Autodesk Fusion 360 part; units mm, degrees
(part 2 of 5)
  spline S372 degree 3 poles (4.7111, -23.5702) (4.7722, -23.6439) (4.9893, -23.6685) (5.5782, -23.6685) knots 0 0 0 0 1 1 1 1
  spline S373 degree 3 poles (5.5782, -23.6685) (6.2377, -23.6685) (6.3816, -23.6488) (6.4743, -23.546) knots 0 0 0 0 1 1 1 1
  spline S374 degree 3 poles (-7.1959, -23.494) (-7.0891, -23.3973) (-7.0889, -23.3561) (-7.1932, -22.9412) knots 0 0 0 0 1 1 1 1
  spline S375 degree 3 poles (-7.1932, -22.9412) (-7.3658, -22.2555) (-7.3564, -22.261) (-8.3356, -22.2838) knots 0 0 0 0 1 1 1 1
  spline S376 degree 3 poles (-8.3356, -22.2838) (-9.3649, -22.3078) (-9.3935, -22.3315) (-9.1564, -22.9655) knots 0 0 0 0 1 1 1 1
  spline S377 degree 3 poles (-9.1564, -22.9655) (-9.0671, -23.2043) (-8.9493, -23.4445) (-8.8946, -23.4991) knots 0 0 0 0 1 1 1 1
  spline S378 degree 3 poles (-8.8946, -23.4991) (-8.7496, -23.6442) (-7.3571, -23.64) (-7.1958, -23.494) knots 0 0 0 0 1 1 1 1
  line L37 (-7.1958, -23.494) -> (-7.1959, -23.494)
  spline S379 degree 3 poles (-9.9736, -23.403) (-9.8682, -23.2865) (-9.8793, -23.2228) (-10.1295, -22.5104) knots 0 0 0 0 1 1 1 1
  spline S380 degree 3 poles (-10.1295, -22.5104) (-10.2776, -22.0885) (-10.4869, -21.4283) (-10.5946, -21.0433) knots 0 0 0 0 1 1 1 1
  spline S381 degree 3 poles (-10.5946, -21.0433) (-10.7023, -20.6583) (-10.8399, -20.2914) (-10.9004, -20.2281) knots 0 0 0 0 1 1 1 1
  spline S382 degree 3 poles (-10.9004, -20.2281) (-10.994, -20.1302) (-11.2635, -20.1058) (-12.6957, -20.0659) knots 0 0 0 0 1 1 1 1
  spline S383 degree 3 poles (-12.6957, -20.0659) (-14.1773, -20.0246) (-14.3919, -20.0322) (-14.4718, -20.1285) knots 0 0 0 0 1 1 1 1
  spline S384 degree 3 poles (-14.4718, -20.1285) (-14.5866, -20.2669) (-14.5722, -20.3045) (-13.7547, -22.0046) knots 0 0 0 0 1 1 1 1
  spline S385 degree 3 poles (-13.7547, -22.0046) (-13.3004, -22.9493) (-13.0832, -23.3288) (-12.9778, -23.3623) knots 0 0 0 0 1 1 1 1
  spline S386 degree 3 poles (-12.9778, -23.3623) (-12.8973, -23.3878) (-12.3588, -23.4307) (-11.781, -23.4576) knots 0 0 0 0 1 1 1 1
  spline S387 degree 3 poles (-11.781, -23.4576) (-10.0405, -23.5385) (-10.0978, -23.5402) (-9.9736, -23.403) knots 0 0 0 0 1 1 1 1
  spline S388 degree 3 poles (-14.1996, -23.1857) (-14.143, -23.08) (-14.2184, -22.8627) (-14.5697, -22.1181) knots 0 0 0 0 1 1 1 1
  spline S389 degree 3 poles (-14.5697, -22.1181) (-14.8124, -21.604) (-15.101, -20.9628) (-15.2112, -20.6933) knots 0 0 0 0 1 1 1 1
  spline S390 degree 3 poles (-15.2112, -20.6933) (-15.4743, -20.0495) (-15.5372, -19.9847) (-15.9461, -19.9363) knots 0 0 0 0 1 1 1 1
  spline S391 degree 3 poles (-15.9461, -19.9363) (-16.4654, -19.8747) (-16.6, -19.7815) (-16.5476, -19.5194) knots 0 0 0 0 1 1 1 1
  spline S392 degree 3 poles (-16.5476, -19.5194) (-16.5238, -19.4006) (-16.4863, -19.2854) (-16.4641, -19.2633) knots 0 0 0 0 1 1 1 1
  spline S393 degree 3 poles (-16.4641, -19.2633) (-16.4419, -19.2412) (-16.0001, -19.221) (-15.4823, -19.2183) knots 0 0 0 0 1 1 1 1
  spline S394 degree 3 poles (-15.4823, -19.2183) (-14.2548, -19.2118) (-14.2482, -19.2065) (-14.5082, -18.4258) knots 0 0 0 0 1 1 1 1
  spline S395 degree 3 poles (-14.5082, -18.4258) (-14.6119, -18.1144) (-14.7295, -17.8393) (-14.7696, -17.8145) knots 0 0 0 0 1 1 1 1
  spline S396 degree 3 poles (-14.7696, -17.8145) (-14.8097, -17.7898) (-15.6499, -17.7301) (-16.6367, -17.6821) knots 0 0 0 0 1 1 1 1
  spline S397 degree 3 poles (-16.6367, -17.6821) (-18.9056, -17.5715) (-18.8123, -17.5261) (-18.3746, -18.5267) knots 0 0 0 0 1 1 1 1
  spline S398 degree 3 poles (-18.3746, -18.5267) (-17.8444, -19.7387) (-17.26, -20.864) (-17.1434, -20.8975) knots 0 0 0 0 1 1 1 1
  spline S399 degree 3 poles (-17.1434, -20.8975) (-17.0815, -20.9152) (-16.8104, -20.9496) (-16.5409, -20.9738) knots 0 0 0 0 1 1 1 1
  spline S400 degree 3 poles (-16.5409, -20.9738) (-15.8303, -21.0378) (-15.6634, -21.1154) (-15.6911, -21.3691) knots 0 0 0 0 1 1 1 1
  spline S401 degree 3 poles (-15.6911, -21.3691) (-15.7208, -21.6402) (-15.7927, -21.7015) (-16.1537, -21.7631) knots 0 0 0 0 1 1 1 1
  spline S402 degree 3 poles (-16.1537, -21.7631) (-16.6452, -21.847) (-16.6576, -21.9608) (-16.2479, -22.631) knots 0 0 0 0 1 1 1 1
  line L38 (-16.2479, -22.631) -> (-15.8919, -23.2134)
  line L39 (-15.8919, -23.2134) -> (-15.5163, -23.2545)
  spline S403 degree 3 poles (-15.5163, -23.2545) (-15.3098, -23.2771) (-14.945, -23.3008) (-14.7057, -23.307) knots 0 0 0 0 1 1 1 1
  spline S404 degree 3 poles (-14.7057, -23.307) (-14.3431, -23.3165) (-14.2588, -23.2963) (-14.1996, -23.1857) knots 0 0 0 0 1 1 1 1
  spline S405 degree 3 poles (-17.102, -22.9718) (-17.059, -22.8365) (-17.5324, -21.8727) (-17.7164, -21.7208) knots 0 0 0 0 1 1 1 1
  spline S406 degree 3 poles (-17.7164, -21.7208) (-17.7629, -21.6824) (-18.1599, -21.6235) (-18.5986, -21.5898) knots 0 0 0 0 1 1 1 1
  spline S407 degree 3 poles (-18.5986, -21.5898) (-19.239, -21.5407) (-19.415, -21.5473) (-19.4912, -21.6235) knots 0 0 0 0 1 1 1 1
  spline S408 degree 3 poles (-19.4912, -21.6235) (-19.6306, -21.7629) (-19.6169, -21.8042) (-19.2605, -22.3212) knots 0 0 0 0 1 1 1 1
  spline S409 degree 3 poles (-19.2605, -22.3212) (-18.7699, -23.0329) (-18.7746, -23.0291) (-18.3356, -23.0569) knots 0 0 0 0 1 1 1 1
  spline S410 degree 3 poles (-18.3356, -23.0569) (-17.272, -23.1244) (-17.1477, -23.1158) (-17.102, -22.9718) knots 0 0 0 0 1 1 1 1
  spline S411 degree 3 poles (-20.085, -22.7052) (-20.0339, -22.6096) (-20.1018, -22.4584) (-20.3884, -22.0305) knots 0 0 0 0 1 1 1 1
  spline S412 degree 3 poles (-20.3884, -22.0305) (-20.5916, -21.7273) (-20.8035, -21.4536) (-20.8592, -21.4224) knots 0 0 0 0 1 1 1 1
  spline S413 degree 3 poles (-20.8592, -21.4224) (-20.915, -21.3912) (-21.3167, -21.3561) (-21.7518, -21.3445) knots 0 0 0 0 1 1 1 1
  spline S414 degree 3 poles (-21.7518, -21.3445) (-22.7883, -21.3168) (-22.836, -21.3702) (-22.3361, -21.9981) knots 0 0 0 0 1 1 1 1
  spline S415 degree 3 poles (-22.3361, -21.9981) (-21.8149, -22.6526) (-21.7425, -22.7033) (-21.2489, -22.7595) knots 0 0 0 0 1 1 1 1
  spline S416 degree 3 poles (-21.2489, -22.7595) (-20.431, -22.8525) (-20.1571, -22.8397) (-20.085, -22.7052) knots 0 0 0 0 1 1 1 1
  spline S417 degree 3 poles (-23.2586, -22.26) (-23.2271, -22.1608) (-23.2597, -22.0505) (-23.3567, -21.9275) knots 0 0 0 0 1 1 1 1
  spline S418 degree 3 poles (-23.3567, -21.9275) (-23.4366, -21.8262) (-23.8688, -21.1996) (-24.3173, -20.5351) knots 0 0 0 0 1 1 1 1
  spline S419 degree 3 poles (-24.3173, -20.5351) (-24.8725, -19.7122) (-25.1802, -19.3178) (-25.282, -19.2986) knots 0 0 0 0 1 1 1 1
  spline S420 degree 3 poles (-25.282, -19.2986) (-25.3642, -19.283) (-25.8252, -19.2171) (-26.3065, -19.152) knots 0 0 0 0 1 1 1 1
  spline S421 degree 3 poles (-26.3065, -19.152) (-26.7877, -19.0869) (-27.2603, -19.0193) (-27.3565, -19.0016) knots 0 0 0 0 1 1 1 1
  spline S422 degree 3 poles (-27.3565, -19.0016) (-27.4814, -18.9787) (-27.5572, -19.0116) (-27.6213, -19.1165) knots 0 0 0 0 1 1 1 1
  spline S423 degree 3 poles (-27.6213, -19.1165) (-27.7025, -19.2494) (-27.6628, -19.3282) (-27.2043, -19.9434) knots 0 0 0 0 1 1 1 1
  spline S424 degree 3 poles (-27.2043, -19.9434) (-26.2552, -21.2168) (-25.7357, -21.7909) (-25.3964, -21.9414) knots 0 0 0 0 1 1 1 1
  spline S425 degree 3 poles (-25.3964, -21.9414) (-25.0384, -22.1001) (-23.8634, -22.389) (-23.5285, -22.4007) knots 0 0 0 0 1 1 1 1
  spline S426 degree 3 poles (-23.5285, -22.4007) (-23.3591, -22.4065) (-23.2944, -22.3728) (-23.2586, -22.26) knots 0 0 0 0 1 1 1 1
  spline S427 degree 3 poles (-18.3724, -20.6471) (-18.3163, -20.5575) (-18.3683, -20.3894) (-18.5996, -19.9121) knots 0 0 0 0 1 1 1 1
  spline S428 degree 3 poles (-18.5996, -19.9121) (-18.7646, -19.5717) (-19.0595, -18.9199) (-19.2549, -18.4637) knots 0 0 0 0 1 1 1 1
  spline S429 degree 3 poles (-19.2549, -18.4637) (-19.499, -17.8936) (-19.6556, -17.6161) (-19.7556, -17.5766) knots 0 0 0 0 1 1 1 1
  spline S430 degree 3 poles (-19.7556, -17.5766) (-19.8356, -17.545) (-20.6729, -17.4756) (-21.6162, -17.4225) knots 0 0 0 0 1 1 1 1
  spline S431 degree 3 poles (-21.6162, -17.4225) (-23.2619, -17.3298) (-23.3369, -17.3312) (-23.4713, -17.4555) knots 0 0 0 0 1 1 1 1
  spline S432 degree 3 poles (-23.4713, -17.4555) (-23.6106, -17.5844) (-23.6096, -17.5883) (-23.2756, -18.2138) knots 0 0 0 0 1 1 1 1
  line L40 (-23.2756, -18.2138) -> (-22.9399, -18.8425)
  line L41 (-22.9399, -18.8425) -> (-23.138, -19.1378)
  spline S433 degree 3 poles (-23.138, -19.1378) (-23.2893, -19.3634) (-23.3917, -19.4415) (-23.5714, -19.4682) knots 0 0 0 0 1 1 1 1
  spline S434 degree 3 poles (-23.5714, -19.4682) (-23.9431, -19.5235) (-23.9843, -19.6738) (-23.7292, -20.0445) knots 0 0 0 0 1 1 1 1
  spline S435 degree 3 poles (-23.7292, -20.0445) (-23.4858, -20.3982) (-23.4696, -20.4032) (-22.2788, -20.4886) knots 0 0 0 0 1 1 1 1
  spline S436 degree 3 poles (-22.2788, -20.4886) (-21.7451, -20.5269) (-21.6317, -20.5163) (-21.5526, -20.421) knots 0 0 0 0 1 1 1 1
  spline S437 degree 3 poles (-21.5526, -20.421) (-21.4724, -20.3244) (-21.4954, -20.2386) (-21.7125, -19.8254) knots 0 0 0 0 1 1 1 1
  spline S438 degree 3 poles (-21.7125, -19.8254) (-22.0273, -19.2265) (-22.0381, -19.019) (-21.7622, -18.8763) knots 0 0 0 0 1 1 1 1
  spline S439 degree 3 poles (-21.7622, -18.8763) (-21.5644, -18.774) (-21.5523, -18.7777) (-21.3568, -19.0003) knots 0 0 0 0 1 1 1 1
  spline S440 degree 3 poles (-21.3568, -19.0003) (-21.246, -19.1265) (-20.9836, -19.535) (-20.7737, -19.9081) knots 0 0 0 0 1 1 1 1
  spline S441 degree 3 poles (-20.7737, -19.9081) (-20.5638, -20.2811) (-20.3446, -20.6075) (-20.2866, -20.6333) knots 0 0 0 0 1 1 1 1
  spline S442 degree 3 poles (-20.2866, -20.6333) (-20.1603, -20.6895) (-19.1029, -20.7825) (-18.7181, -20.7713) knots 0 0 0 0 1 1 1 1
  spline S443 degree 3 poles (-18.7181, -20.7713) (-18.5465, -20.7662) (-18.4182, -20.7202) (-18.3724, -20.6471) knots 0 0 0 0 1 1 1 1
  spline S444 degree 3 poles (-11.2586, -19.227) (-11.1806, -19.1329) (-11.2075, -18.9413) (-11.4286, -18.0142) knots 0 0 0 0 1 1 1 1
  spline S445 degree 3 poles (-11.4286, -18.0142) (-11.8311, -16.3265) (-11.8724, -16.1679) (-11.9215, -16.1187) knots 0 0 0 0 1 1 1 1
  spline S446 degree 3 poles (-11.9215, -16.1187) (-11.9465, -16.0936) (-12.4728, -16.073) (-13.0908, -16.073) knots 0 0 0 0 1 1 1 1
  spline S447 degree 3 poles (-13.0908, -16.073) (-14.0289, -16.073) (-14.2259, -16.0909) (-14.2834, -16.1814) knots 0 0 0 0 1 1 1 1
  spline S448 degree 3 poles (-14.2834, -16.1814) (-14.333, -16.2596) (-14.2415, -16.6488) (-13.9539, -17.5815) knots 0 0 0 0 1 1 1 1
  spline S449 degree 3 poles (-13.9539, -17.5815) (-13.7348, -18.2919) (-13.5182, -18.9519) (-13.4725, -19.0482) knots 0 0 0 0 1 1 1 1
  spline S450 degree 3 poles (-13.4725, -19.0482) (-13.376, -19.2514) (-13.222, -19.2813) (-12.091, -19.3159) knots 0 0 0 0 1 1 1 1
  spline S451 degree 3 poles (-12.091, -19.3159) (-11.4803, -19.3346) (-11.3351, -19.3191) (-11.2586, -19.227) knots 0 0 0 0 1 1 1 1
  spline S452 degree 3 poles (12.1431, -19.1357) (12.2424, -19.0239) (12.8257, -17.0786) (12.9356, -16.4928) knots 0 0 0 0 1 1 1 1
  spline S453 degree 3 poles (12.9356, -16.4928) (13.006, -16.1179) (12.8869, -16.0228) (12.3751, -16.0451) knots 0 0 0 0 1 1 1 1
  spline S454 degree 3 poles (12.3751, -16.0451) (12.1418, -16.0553) (11.8485, -16.0396) (11.7234, -16.0103) knots 0 0 0 0 1 1 1 1
  spline S455 degree 3 poles (11.7234, -16.0103) (11.522, -15.963) (11.4959, -15.9296) (11.4959, -15.7199) knots 0 0 0 0 1 1 1 1
  spline S456 degree 3 poles (11.4959, -15.7199) (11.4959, -15.5464) (11.5377, -15.4605) (11.652, -15.3993) knots 0 0 0 0 1 1 1 1
  spline S457 degree 3 poles (11.652, -15.3993) (11.8021, -15.319) (11.9349, -15.3043) (12.7335, -15.2793) knots 0 0 0 0 1 1 1 1
  spline S458 degree 3 poles (12.7335, -15.2793) (12.9329, -15.273) (13.1376, -15.2262) (13.1885, -15.1751) knots 0 0 0 0 1 1 1 1
  spline S459 degree 3 poles (13.1885, -15.1751) (13.2746, -15.0887) (13.4125, -14.5028) (13.7235, -12.9022) knots 0 0 0 0 1 1 1 1
  spline S460 degree 3 poles (13.7235, -12.9022) (13.9057, -11.9647) (13.9654, -12.0047) (12.4467, -12.0477) knots 0 0 0 0 1 1 1 1
  spline S461 degree 3 poles (12.4467, -12.0477) (11.5543, -12.073) (11.1952, -12.1075) (11.1556, -12.1717) knots 0 0 0 0 1 1 1 1
  spline S462 degree 3 poles (11.1556, -12.1717) (11.1255, -12.2205) (11.0293, -12.7561) (10.9418, -13.3617) knots 0 0 0 0 1 1 1 1
  spline S463 degree 3 poles (10.9418, -13.3617) (10.7112, -14.9572) (10.5495, -15.892) (10.2268, -17.4942) knots 0 0 0 0 1 1 1 1
  spline S464 degree 3 poles (10.2268, -17.4942) (9.8688, -19.2718) (9.8248, -19.1742) (10.9973, -19.206) knots 0 0 0 0 1 1 1 1
  spline S465 degree 3 poles (10.9973, -19.206) (11.4448, -19.2181) (11.8612, -19.2349) (11.9226, -19.2431) knots 0 0 0 0 1 1 1 1
  spline S466 degree 3 poles (11.9226, -19.2431) (11.984, -19.2514) (12.0832, -19.2031) (12.1431, -19.1357) knots 0 0 0 0 1 1 1 1
  spline S467 degree 3 poles (9.0635, -18.9957) (9.2364, -18.8023) (10.0525, -14.4881) (10.274, -12.5966) knots 0 0 0 0 1 1 1 1
  spline S468 degree 3 poles (10.274, -12.5966) (10.3165, -12.2337) (10.3072, -12.1934) (10.1633, -12.1164) knots 0 0 0 0 1 1 1 1
  spline S469 degree 3 poles (10.1633, -12.1164) (10.045, -12.0531) (9.4611, -12.0445) (7.7934, -12.0813) knots 0 0 0 0 1 1 1 1
  line L42 (7.7934, -12.0813) -> (5.5805, -12.1302)
  line L43 (5.5805, -12.1302) -> (5.3302, -11.8614)
  line L44 (5.3302, -11.8614) -> (5.0798, -11.5927)
  line L45 (5.0798, -11.5927) -> (5.1304, -10.7527)
  spline S470 degree 3 poles (5.1304, -10.7527) (5.1909, -9.7502) (5.1532, -9.6653) (4.6609, -9.6943) knots 0 0 0 0 1 1 1 1
  spline S471 degree 3 poles (4.6609, -9.6943) (4.4902, -9.7044) (4.3075, -9.7576) (4.2549, -9.8126) knots 0 0 0 0 1 1 1 1
  spline S472 degree 3 poles (4.2549, -9.8126) (4.1902, -9.8804) (4.1457, -10.1938) (4.1167, -10.7851) knots 0 0 0 0 1 1 1 1
  spline S473 degree 3 poles (4.1167, -10.7851) (4.0745, -11.6468) (4.0712, -11.6604) (3.851, -11.8876) knots 0 0 0 0 1 1 1 1
  line L46 (3.851, -11.8876) -> (3.6279, -12.1178)
  line L47 (3.6279, -12.1178) -> (1.9108, -12.1178)
  line L48 (1.9108, -12.1178) -> (0.1937, -12.1178)
  line L49 (0.1937, -12.1178) -> (-0.0377, -11.8576)
  line L50 (-0.0377, -11.8576) -> (-0.2692, -11.5974)
  line L51 (-0.2692, -11.5974) -> (-0.2623, -9.9278)
  spline S474 degree 3 poles (-0.2623, -9.9278) (-0.2573, -8.7307) (-0.2789, -8.2299) (-0.3387, -8.1579) knots 0 0 0 0 1 1 1 1
  spline S475 degree 3 poles (-0.3387, -8.1579) (-0.392, -8.0936) (-0.5566, -8.0575) (-0.796, -8.0575) knots 0 0 0 0 1 1 1 1
  spline S476 degree 3 poles (-0.796, -8.0575) (-1.323, -8.0575) (-1.3327, -8.0876) (-1.2858, -9.5846) knots 0 0 0 0 1 1 1 1
  spline S477 degree 3 poles (-1.2858, -9.5846) (-1.2645, -10.2655) (-1.2272, -11.813) (-1.2029, -13.0234) knots 0 0 0 0 1 1 1 1
  spline S478 degree 3 poles (-1.2029, -13.0234) (-1.1693, -14.6996) (-1.1368, -15.246) (-1.0668, -15.316) knots 0 0 0 0 1 1 1 1
  spline S479 degree 3 poles (-1.0668, -15.316) (-0.9937, -15.3891) (-0.3524, -15.408) (2.0616, -15.408) knots 0 0 0 0 1 1 1 1
  line L52 (2.0616, -15.408) -> (5.098, -15.408)
  line L53 (5.098, -15.408) -> (5.3267, -15.6439)
  line L54 (5.3267, -15.6439) -> (5.5554, -15.8799)
  line L55 (5.5554, -15.8799) -> (5.449, -16.8515)
  spline S480 degree 3 poles (5.449, -16.8515) (5.3904, -17.3859) (5.3225, -18.0465) (5.298, -18.3196) knots 0 0 0 0 1 1 1 1
  spline S481 degree 3 poles (5.298, -18.3196) (5.2336, -19.0388) (5.2487, -19.0484) (6.4431, -19.0471) knots 0 0 0 0 1 1 1 1
  spline S482 degree 3 poles (6.4431, -19.0471) (6.9697, -19.0466) (7.4397, -19.0213) (7.4873, -18.991) knots 0 0 0 0 1 1 1 1
  spline S483 degree 3 poles (7.4873, -18.991) (7.5828, -18.9303) (7.6234, -18.7423) (7.9279, -16.948) knots 0 0 0 0 1 1 1 1
  spline S484 degree 3 poles (7.9279, -16.948) (8.0422, -16.2743) (8.1725, -15.6331) (8.2173, -15.5232) knots 0 0 0 0 1 1 1 1
  spline S485 degree 3 poles (8.2173, -15.5232) (8.2902, -15.3443) (8.3241, -15.3275) (8.5409, -15.3627) knots 0 0 0 0 1 1 1 1
  spline S486 degree 3 poles (8.5409, -15.3627) (8.6741, -15.3843) (8.796, -15.4149) (8.8118, -15.4307) knots 0 0 0 0 1 1 1 1
  spline S487 degree 3 poles (8.8118, -15.4307) (8.8949, -15.5138) (8.8285, -16.227) (8.6205, -17.4874) knots 0 0 0 0 1 1 1 1
  spline S488 degree 3 poles (8.6205, -17.4874) (8.4259, -18.6659) (8.4031, -18.9136) (8.4804, -19.0068) knots 0 0 0 0 1 1 1 1
  spline S489 degree 3 poles (8.4804, -19.0068) (8.6032, -19.1548) (8.9269, -19.1486) (9.0635, -18.9957) knots 0 0 0 0 1 1 1 1
  spline S490 degree 3 poles (4.4068, -18.8907) (4.4445, -18.8425) (4.5318, -18.2608) (4.6008, -17.5979) knots 0 0 0 0 1 1 1 1
  spline S491 degree 3 poles (4.6008, -17.5979) (4.7028, -16.6191) (4.7096, -16.3724) (4.6373, -16.2853) knots 0 0 0 0 1 1 1 1
  spline S492 degree 3 poles (4.6373, -16.2853) (4.5614, -16.1938) (4.2703, -16.178) (2.6548, -16.178) knots 0 0 0 0 1 1 1 1
  spline S493 degree 3 poles (2.6548, -16.178) (0.9911, -16.178) (0.7457, -16.1921) (0.6332, -16.2939) knots 0 0 0 0 1 1 1 1
  spline S494 degree 3 poles (0.6332, -16.2939) (0.519, -16.3972) (0.5052, -16.5347) (0.5052, -17.5659) knots 0 0 0 0 1 1 1 1
  spline S495 degree 3 poles (0.5052, -17.5659) (0.5052, -18.5436) (0.5231, -18.7419) (0.6211, -18.8502) knots 0 0 0 0 1 1 1 1
  spline S496 degree 3 poles (0.6211, -18.8502) (0.7276, -18.9679) (0.882, -18.9782) (2.5376, -18.9782) knots 0 0 0 0 1 1 1 1
  spline S497 degree 3 poles (2.5376, -18.9782) (3.895, -18.9782) (4.3552, -18.9566) (4.4068, -18.8907) knots 0 0 0 0 1 1 1 1
  spline S498 degree 3 poles (-24.1816, -18.4751) (-24.1231, -18.3818) (-24.2127, -18.1392) (-24.6081, -17.32) knots 0 0 0 0 1 1 1 1
  spline S499 degree 3 poles (-24.6081, -17.32) (-25.2286, -16.0342) (-25.3784, -15.693) (-25.8625, -14.4629) knots 0 0 0 0 1 1 1 1
  spline S500 degree 3 poles (-25.8625, -14.4629) (-26.0747, -13.9239) (-26.2692, -13.4619) (-26.2949, -13.4362) knots 0 0 0 0 1 1 1 1
  spline S501 degree 3 poles (-26.2949, -13.4362) (-26.3205, -13.4106) (-26.4578, -13.3717) (-26.6, -13.3497) knots 0 0 0 0 1 1 1 1
  spline S502 degree 3 poles (-26.6, -13.3497) (-26.8567, -13.3101) (-27.0765, -13.4258) (-27.0765, -13.6005) knots 0 0 0 0 1 1 1 1
  spline S503 degree 3 poles (-27.0765, -13.6005) (-27.0765, -13.9542) (-25.0421, -18.052) (-24.6397, -18.5087) knots 0 0 0 0 1 1 1 1
  spline S504 degree 3 poles (-24.6397, -18.5087) (-24.5088, -18.6573) (-24.2856, -18.6409) (-24.1816, -18.4751) knots 0 0 0 0 1 1 1 1
  spline S505 degree 3 poles (-25.8887, -18.2823) (-25.829, -18.1709) (-25.9369, -17.9059) (-26.489, -16.8075) knots 0 0 0 0 1 1 1 1
  spline S506 degree 3 poles (-26.489, -16.8075) (-26.9613, -15.868) (-27.2067, -15.4523) (-27.3118, -15.414) knots 0 0 0 0 1 1 1 1
  spline S507 degree 3 poles (-27.3118, -15.414) (-27.3941, -15.384) (-27.8735, -15.321) (-28.377, -15.274) knots 0 0 0 0 1 1 1 1
  spline S508 degree 3 poles (-28.377, -15.274) (-28.8806, -15.2271) (-29.4161, -15.1605) (-29.5671, -15.1262) knots 0 0 0 0 1 1 1 1
  spline S509 degree 3 poles (-29.5671, -15.1262) (-29.794, -15.0746) (-29.864, -15.086) (-29.9707, -15.1918) knots 0 0 0 0 1 1 1 1
  spline S510 degree 3 poles (-29.9707, -15.1918) (-30.1248, -15.3448) (-30.1463, -15.2948) (-29.2984, -16.7621) knots 0 0 0 0 1 1 1 1
  spline S511 degree 3 poles (-29.2984, -16.7621) (-28.9106, -17.4333) (-28.6715, -17.7719) (-28.5207, -17.8636) knots 0 0 0 0 1 1 1 1
  spline S512 degree 3 poles (-28.5207, -17.8636) (-28.3038, -17.9955) (-27.7635, -18.1352) (-26.7855, -18.3124) knots 0 0 0 0 1 1 1 1
  spline S513 degree 3 poles (-26.7855, -18.3124) (-26.0731, -18.4414) (-25.972, -18.4381) (-25.8887, -18.2823) knots 0 0 0 0 1 1 1 1
  spline S514 degree 3 poles (-0.3274, -17.3241) (-0.2168, -17.1909) (-0.2326, -16.4063) (-0.3486, -16.2665) knots 0 0 0 0 1 1 1 1
  spline S515 degree 3 poles (-0.3486, -16.2665) (-0.4019, -16.2022) (-0.7155, -16.178) (-1.4935, -16.178) knots 0 0 0 0 1 1 1 1
  spline S516 degree 3 poles (-1.4935, -16.178) (-2.777, -16.178) (-2.7946, -16.1867) (-2.7355, -16.7905) knots 0 0 0 0 1 1 1 1
  spline S517 degree 3 poles (-2.7355, -16.7905) (-2.7138, -17.0119) (-2.6662, -17.231) (-2.6297, -17.2773) knots 0 0 0 0 1 1 1 1
  spline S518 degree 3 poles (-2.6297, -17.2773) (-2.559, -17.367) (-2.1789, -17.4036) (-1.096, -17.4249) knots 0 0 0 0 1 1 1 1
  spline S519 degree 3 poles (-1.096, -17.4249) (-0.5475, -17.4356) (-0.4044, -17.4169) (-0.3274, -17.3241) knots 0 0 0 0 1 1 1 1
  spline S520 degree 3 poles (-6.8492, -17.2678) (-6.7343, -17.1294) (-6.8029, -16.4006) (-6.9441, -16.2593) knots 0 0 0 0 1 1 1 1
  spline S521 degree 3 poles (-6.9441, -16.2593) (-7.0009, -16.2024) (-7.2534, -16.1552) (-7.586, -16.1392) knots 0 0 0 0 1 1 1 1
  spline S522 degree 3 poles (-7.586, -16.1392) (-8.1756, -16.1109) (-8.476, -15.9692) (-8.5896, -15.6658) knots 0 0 0 0 1 1 1 1
  spline S523 degree 3 poles (-8.5896, -15.6658) (-8.621, -15.5817) (-8.735, -14.7884) (-8.8428, -13.9029) knots 0 0 0 0 1 1 1 1
  spline S524 degree 3 poles (-8.8428, -13.9029) (-8.9747, -12.8194) (-9.0729, -12.2527) (-9.143, -12.1703) knots 0 0 0 0 1 1 1 1
  spline S525 degree 3 poles (-9.143, -12.1703) (-9.2687, -12.0223) (-9.7019, -12.0062) (-9.8884, -12.1426) knots 0 0 0 0 1 1 1 1
  spline S526 degree 3 poles (-9.8884, -12.1426) (-10.0098, -12.2314) (-10.0126, -12.2795) (-9.9317, -12.8952) knots 0 0 0 0 1 1 1 1
  spline S527 degree 3 poles (-9.9317, -12.8952) (-9.7587, -14.2118) (-9.2462, -17.1551) (-9.1773, -17.2277) knots 0 0 0 0 1 1 1 1
  spline S528 degree 3 poles (-9.1773, -17.2277) (-9.1327, -17.2747) (-8.4963, -17.3282) (-7.6463, -17.3565) knots 0 0 0 0 1 1 1 1
  spline S529 degree 3 poles (-7.6463, -17.3565) (-7.0666, -17.3757) (-6.9257, -17.3601) (-6.8492, -17.2678) knots 0 0 0 0 1 1 1 1
  spline S530 degree 3 poles (-3.5541, -17.262) (-3.4519, -17.1388) (-3.511, -16.4205) (-3.6357, -16.2701) knots 0 0 0 0 1 1 1 1
  spline S531 degree 3 poles (-3.6357, -16.2701) (-3.6864, -16.2091) (-3.8923, -16.1773) (-4.2462, -16.176) knots 0 0 0 0 1 1 1 1
  spline S532 degree 3 poles (-4.2462, -16.176) (-4.7417, -16.1741) (-4.797, -16.1586) (-5.0143, -15.961) knots 0 0 0 0 1 1 1 1
  spline S533 degree 3 poles (-5.0143, -15.961) (-5.2746, -15.7243) (-5.2587, -15.8226) (-5.4438, -13.3131) knots 0 0 0 0 1 1 1 1
  spline S534 degree 3 poles (-5.4438, -13.3131) (-5.4848, -12.7577) (-5.553, -12.2616) (-5.5953, -12.2106) knots 0 0 0 0 1 1 1 1
  spline S535 degree 3 poles (-5.5953, -12.2106) (-5.7007, -12.0835) (-6.3143, -12.0891) (-6.4213, -12.2181) knots 0 0 0 0 1 1 1 1
  spline S536 degree 3 poles (-6.4213, -12.2181) (-6.5158, -12.3319) (-6.5011, -12.5475) (-6.2418, -14.848) knots 0 0 0 0 1 1 1 1
  spline S537 degree 3 poles (-6.2418, -14.848) (-6.1485, -15.6758) (-6.0523, -16.5367) (-6.0281, -16.7611) knots 0 0 0 0 1 1 1 1
  spline S538 degree 3 poles (-6.0281, -16.7611) (-6.0039, -16.9856) (-5.9393, -17.214) (-5.8846, -17.2687) knots 0 0 0 0 1 1 1 1
  spline S539 degree 3 poles (-5.8846, -17.2687) (-5.7347, -17.4186) (-3.6792, -17.4127) (-3.5541, -17.262) knots 0 0 0 0 1 1 1 1
  spline S540 degree 3 poles (-15.1066, -16.8441) (-15.037, -16.7602) (-15.0743, -16.5346) (-15.3008, -15.6716) knots 0 0 0 0 1 1 1 1
  spline S541 degree 3 poles (-15.3008, -15.6716) (-15.6004, -14.5299) (-15.7929, -13.7041) (-15.9825, -12.7478) knots 0 0 0 0 1 1 1 1
  spline S542 degree 3 poles (-15.9825, -12.7478) (-16.0474, -12.4205) (-16.1325, -12.1134) (-16.1717, -12.0653) knots 0 0 0 0 1 1 1 1
  spline S543 degree 3 poles (-16.1717, -12.0653) (-16.2109, -12.0171) (-16.3928, -11.9778) (-16.5759, -11.9778) knots 0 0 0 0 1 1 1 1
  spline S544 degree 3 poles (-16.5759, -11.9778) (-17.1125, -11.9778) (-17.1272, -12.038) (-16.8577, -13.1358) knots 0 0 0 0 1 1 1 1
  line L56 (-16.8577, -13.1358) -> (-16.6267, -14.077)
  line L57 (-16.6267, -14.077) -> (-16.8123, -14.3575)
  line L58 (-16.8123, -14.3575) -> (-16.9979, -14.6379)
  line L59 (-16.9979, -14.6379) -> (-17.8029, -14.6379)
  line L60 (-17.8029, -14.6379) -> (-18.608, -14.6379)
  line L61 (-18.608, -14.6379) -> (-18.8503, -14.4104)
  spline S545 degree 3 poles (-18.8503, -14.4104) (-19.0511, -14.2219) (-19.1284, -14.0569) (-19.3011, -13.4479) knots 0 0 0 0 1 1 1 1
  spline S546 degree 3 poles (-19.3011, -13.4479) (-19.4157, -13.0436) (-19.5438, -12.5578) (-19.5858, -12.3683) knots 0 0 0 0 1 1 1 1
  spline S547 degree 3 poles (-19.5858, -12.3683) (-19.6277, -12.1789) (-19.7158, -11.983) (-19.7815, -11.933) knots 0 0 0 0 1 1 1 1
  spline S548 degree 3 poles (-19.7815, -11.933) (-19.9591, -11.7981) (-22.1975, -11.7997) (-22.3096, -11.9349) knots 0 0 0 0 1 1 1 1
  spline S549 degree 3 poles (-22.3096, -11.9349) (-22.4024, -12.0467) (-22.2399, -12.6655) (-21.7124, -14.2095) knots 0 0 0 0 1 1 1 1
  line L62 (-21.7124, -14.2095) -> (-21.3924, -15.1462)
  line L63 (-21.3924, -15.1462) -> (-21.5959, -15.4346)
  spline S550 degree 3 poles (-21.5959, -15.4346) (-21.8297, -15.7659) (-21.7429, -15.7542) (-23.3094, -15.6652) knots 0 0 0 0 1 1 1 1
  spline S551 degree 3 poles (-23.3094, -15.6652) (-24.2304, -15.6129) (-24.2705, -15.6164) (-24.3439, -15.7534) knots 0 0 0 0 1 1 1 1
  spline S552 degree 3 poles (-24.3439, -15.7534) (-24.404, -15.8658) (-24.3894, -15.9565) (-24.2751, -16.1805) knots 0 0 0 0 1 1 1 1
  spline S553 degree 3 poles (-24.2751, -16.1805) (-24.1953, -16.3369) (-24.092, -16.4778) (-24.0457, -16.4935) knots 0 0 0 0 1 1 1 1
  spline S554 degree 3 poles (-24.0457, -16.4935) (-23.9993, -16.5092) (-23.1308, -16.5738) (-22.1158, -16.6371) knots 0 0 0 0 1 1 1 1
  spline S555 degree 3 poles (-22.1158, -16.6371) (-19.88, -16.7766) (-19.9522, -16.7987) (-20.2065, -16.0518) knots 0 0 0 0 1 1 1 1
  spline S556 degree 3 poles (-20.2065, -16.0518) (-20.4111, -15.4508) (-20.3887, -15.1963) (-20.12, -15.0681) knots 0 0 0 0 1 1 1 1
  spline S557 degree 3 poles (-20.12, -15.0681) (-19.9306, -14.9777) (-19.9095, -14.9837) (-19.755, -15.1726) knots 0 0 0 0 1 1 1 1
  spline S558 degree 3 poles (-19.755, -15.1726) (-19.6648, -15.2828) (-19.5899, -15.4052) (-19.5886, -15.4446) knots 0 0 0 0 1 1 1 1
  spline S559 degree 3 poles (-19.5886, -15.4446) (-19.5838, -15.5801) (-19.1577, -16.6332) (-19.0744, -16.7153) knots 0 0 0 0 1 1 1 1
  spline S560 degree 3 poles (-19.0744, -16.7153) (-18.9865, -16.802) (-17.3603, -16.9184) (-15.9719, -16.9374) knots 0 0 0 0 1 1 1 1
  spline S561 degree 3 poles (-15.9719, -16.9374) (-15.3588, -16.9458) (-15.1745, -16.926) (-15.1066, -16.8442) knots 0 0 0 0 1 1 1 1
  line L64 (-15.1066, -16.8442) -> (-15.1066, -16.8441)
  spline S562 degree 3 poles (-7.0248, -15.2052) (-6.9509, -15.0858) (-7.277, -12.2973) (-7.3772, -12.1914) knots 0 0 0 0 1 1 1 1
  spline S563 degree 3 poles (-7.3772, -12.1914) (-7.5231, -12.0371) (-8.0024, -12.0354) (-8.1411, -12.1887) knots 0 0 0 0 1 1 1 1
  spline S564 degree 3 poles (-8.1411, -12.1887) (-8.2433, -12.3015) (-8.2473, -12.393) (-8.1773, -13.0043) knots 0 0 0 0 1 1 1 1
  spline S565 degree 3 poles (-8.1773, -13.0043) (-8.0678, -13.96) (-7.8861, -15.2273) (-7.8538, -15.2614) knots 0 0 0 0 1 1 1 1
  spline S566 degree 3 poles (-7.8538, -15.2614) (-7.839, -15.277) (-7.7084, -15.3109) (-7.5636, -15.3367) knots 0 0 0 0 1 1 1 1
  spline S567 degree 3 poles (-7.5636, -15.3367) (-7.3081, -15.3823) (-7.1033, -15.3323) (-7.0248, -15.2052) knots 0 0 0 0 1 1 1 1
  spline S568 degree 3 poles (-2.0133, -15.301) (-1.944, -15.2175) (-1.9343, -14.7845) (-1.9692, -13.3234) knots 0 0 0 0 1 1 1 1
  spline S569 degree 3 poles (-1.9692, -13.3234) (-1.9938, -12.2945) (-2.0337, -10.2557) (-2.0578, -8.7926) knots 0 0 0 0 1 1 1 1
  spline S570 degree 3 poles (-2.0578, -8.7926) (-2.0934, -6.6395) (-2.1206, -6.1124) (-2.2008, -6.0274) knots 0 0 0 0 1 1 1 1
  spline S571 degree 3 poles (-2.2008, -6.0274) (-2.2846, -5.9387) (-2.6413, -5.9214) (-4.5016, -5.9158) knots 0 0 0 0 1 1 1 1
  spline S572 degree 3 poles (-4.5016, -5.9158) (-7.1033, -5.908) (-6.9539, -5.8616) (-6.8759, -6.6534) knots 0 0 0 0 1 1 1 1
  spline S573 degree 3 poles (-6.8759, -6.6534) (-6.8388, -7.029) (-6.7955, -7.1692) (-6.7006, -7.22) knots 0 0 0 0 1 1 1 1
  spline S574 degree 3 poles (-6.7006, -7.22) (-6.6306, -7.2574) (-5.889, -7.2875) (-5.0343, -7.2875) knots 0 0 0 0 1 1 1 1
  spline S575 degree 3 poles (-5.0343, -7.2875) (-4.1872, -7.2875) (-3.4134, -7.3182) (-3.3146, -7.3557) knots 0 0 0 0 1 1 1 1
  spline S576 degree 3 poles (-3.3146, -7.3557) (-3.17, -7.4107) (-3.135, -7.4708) (-3.135, -7.6639) knots 0 0 0 0 1 1 1 1
  spline S577 degree 3 poles (-3.135, -7.6639) (-3.135, -7.8701) (-3.166, -7.9146) (-3.3555, -7.9807) knots 0 0 0 0 1 1 1 1
  spline S578 degree 3 poles (-3.3555, -7.9807) (-3.4767, -8.0229) (-3.8509, -8.0575) (-4.187, -8.0575) knots 0 0 0 0 1 1 1 1
  spline S579 degree 3 poles (-4.187, -8.0575) (-4.6494, -8.0575) (-4.8195, -8.0835) (-4.8867, -8.1644) knots 0 0 0 0 1 1 1 1
  spline S580 degree 3 poles (-4.8867, -8.1644) (-4.985, -8.2828) (-4.9772, -8.5021) (-4.7431, -12.2228) knots 0 0 0 0 1 1 1 1
  spline S581 degree 3 poles (-4.7431, -12.2228) (-4.5768, -14.8659) (-4.5435, -15.1795) (-4.4155, -15.3075) knots 0 0 0 0 1 1 1 1
  spline S582 degree 3 poles (-4.4155, -15.3075) (-4.2638, -15.4592) (-2.1399, -15.4535) (-2.0133, -15.301) knots 0 0 0 0 1 1 1 1
  spline S583 degree 3 poles (-13.8969, -15.1455) (-13.7958, -15.0333) (-13.8104, -14.9016) (-14.0694, -13.5879) knots 0 0 0 0 1 1 1 1
  spline S584 degree 3 poles (-14.0694, -13.5879) (-14.225, -12.7986) (-14.384, -12.1134) (-14.4226, -12.0653) knots 0 0 0 0 1 1 1 1
  spline S585 degree 3 poles (-14.4226, -12.0653) (-14.5309, -11.9304) (-15.0639, -11.9555) (-15.1961, -12.1016) knots 0 0 0 0 1 1 1 1
  spline S586 degree 3 poles (-15.1961, -12.1016) (-15.2992, -12.2155) (-15.2945, -12.2901) (-15.1374, -13.0292) knots 0 0 0 0 1 1 1 1
  spline S587 degree 3 poles (-15.1374, -13.0292) (-14.8517, -14.373) (-14.6769, -15.0169) (-14.5628, -15.1455) knots 0 0 0 0 1 1 1 1
  spline S588 degree 3 poles (-14.5628, -15.1455) (-14.5021, -15.2138) (-14.3553, -15.268) (-14.2307, -15.268) knots 0 0 0 0 1 1 1 1
  spline S589 degree 3 poles (-14.2307, -15.268) (-14.1068, -15.268) (-13.9582, -15.2134) (-13.8969, -15.1455) knots 0 0 0 0 1 1 1 1
  spline S590 degree 3 poles (14.8771, -15.1436) (14.9405, -15.0735) (15.1275, -14.4091) (15.3049, -13.6232) knots 0 0 0 0 1 1 1 1
  spline S591 degree 3 poles (15.3049, -13.6232) (15.5997, -12.3177) (15.6127, -12.219) (15.5043, -12.0993) knots 0 0 0 0 1 1 1 1
  spline S592 degree 3 poles (15.5043, -12.0993) (15.4179, -12.0038) (15.3083, -11.9766) (15.0721, -11.9921) knots 0 0 0 0 1 1 1 1
  spline S593 degree 3 poles (15.0721, -11.9921) (14.8143, -12.0091) (14.7401, -12.0453) (14.6717, -12.1879) knots 0 0 0 0 1 1 1 1
  spline S594 degree 3 poles (14.6717, -12.1879) (14.5136, -12.5179) (14.0846, -14.9947) (14.1609, -15.1372) knots 0 0 0 0 1 1 1 1
  spline S595 degree 3 poles (14.1609, -15.1372) (14.2549, -15.3128) (14.7202, -15.3169) (14.8771, -15.1436) knots 0 0 0 0 1 1 1 1
  spline S596 degree 3 poles (16.6304, -15.0406) (16.684, -14.954) (16.8761, -14.2739) (17.0573, -13.5293) knots 0 0 0 0 1 1 1 1
  spline S597 degree 3 poles (17.0573, -13.5293) (17.3551, -12.3055) (17.3764, -12.1642) (17.2795, -12.0571) knots 0 0 0 0 1 1 1 1
  spline S598 degree 3 poles (17.2795, -12.0571) (17.1525, -11.9167) (16.633, -11.9202) (16.4936, -12.0622) knots 0 0 0 0 1 1 1 1
  spline S599 degree 3 poles (16.4936, -12.0622) (16.4447, -12.1121) (16.2774, -12.7456) (16.1217, -13.47) knots 0 0 0 0 1 1 1 1
  spline S600 degree 3 poles (16.1217, -13.47) (15.9661, -14.1945) (15.8214, -14.8154) (15.8001, -14.8498) knots 0 0 0 0 1 1 1 1
  spline S601 degree 3 poles (15.8001, -14.8498) (15.7788, -14.8842) (15.8014, -14.9767) (15.8506, -15.0552) knots 0 0 0 0 1 1 1 1
  spline S602 degree 3 poles (15.8506, -15.0552) (15.9829, -15.267) (16.4963, -15.2573) (16.6304, -15.0406) knots 0 0 0 0 1 1 1 1
  spline S603 degree 3 poles (18.3023, -15.0056) (18.3616, -14.9382) (18.5549, -14.3633) (18.7319, -13.728) knots 0 0 0 0 1 1 1 1
  spline S604 degree 3 poles (18.7319, -13.728) (19.1434, -12.2512) (19.1639, -12.1425) (19.0565, -12.0131) knots 0 0 0 0 1 1 1 1
  spline S605 degree 3 poles (19.0565, -12.0131) (18.9317, -11.8627) (18.4063, -11.8743) (18.2747, -12.0304) knots 0 0 0 0 1 1 1 1
  spline S606 degree 3 poles (18.2747, -12.0304) (18.2178, -12.0978) (18.0208, -12.776) (17.8369, -13.5375) knots 0 0 0 0 1 1 1 1
  spline S607 degree 3 poles (17.8369, -13.5375) (17.5684, -14.6491) (17.5193, -14.9425) (17.588, -15.0251) knots 0 0 0 0 1 1 1 1
  spline S608 degree 3 poles (17.588, -15.0251) (17.708, -15.1698) (18.169, -15.1572) (18.3023, -15.0056) knots 0 0 0 0 1 1 1 1
  spline S609 degree 3 poles (-22.4579, -14.7813) (-22.4015, -14.6759) (-22.4342, -14.4958) (-22.6003, -13.9959) knots 0 0 0 0 1 1 1 1
  spline S610 degree 3 poles (-22.6003, -13.9959) (-23.1112, -12.4581) (-23.4709, -11.0999) (-23.8572, -9.2501) knots 0 0 0 0 1 1 1 1
  spline S611 degree 3 poles (-23.8572, -9.2501) (-24.0381, -8.3838) (-24.1645, -7.9302) (-24.2402, -7.8748) knots 0 0 0 0 1 1 1 1
  spline S612 degree 3 poles (-24.2402, -7.8748) (-24.4196, -7.7436) (-26.8204, -7.7427) (-26.9292, -7.8738) knots 0 0 0 0 1 1 1 1
  spline S613 degree 3 poles (-26.9292, -7.8738) (-27.0866, -8.0635) (-26.2634, -11.1168) (-25.4546, -13.343) knots 0 0 0 0 1 1 1 1
  spline S614 degree 3 poles (-25.4546, -13.343) (-25.062, -14.4239) (-24.9503, -14.6719) (-24.8194, -14.755) knots 0 0 0 0 1 1 1 1
  spline S615 degree 3 poles (-24.8194, -14.755) (-24.7291, -14.8122) (-23.8375, -14.8866) (-23.0012, -14.9068) knots 0 0 0 0 1 1 1 1
  spline S616 degree 3 poles (-23.0012, -14.9068) (-22.5997, -14.9164) (-22.5205, -14.8981) (-22.4579, -14.7813) knots 0 0 0 0 1 1 1 1
  spline S617 degree 3 poles (-27.7547, -14.4426) (-27.6494, -14.3262) (-27.6544, -14.2841) (-27.8239, -13.865) knots 0 0 0 0 1 1 1 1
  spline S618 degree 3 poles (-27.8239, -13.865) (-28.3185, -12.6417) (-28.7566, -11.3262) (-28.7566, -11.0643) knots 0 0 0 0 1 1 1 1
  spline S619 degree 3 poles (-28.7566, -11.0643) (-28.7566, -10.9026) (-28.7139, -10.8546) (-28.5101, -10.7873) knots 0 0 0 0 1 1 1 1
  spline S620 degree 3 poles (-28.5101, -10.7873) (-28.2854, -10.7132) (-28.2517, -10.7204) (-28.1292, -10.8694) knots 0 0 0 0 1 1 1 1
  spline S621 degree 3 poles (-28.1292, -10.8694) (-28.0553, -10.9593) (-27.9116, -11.3006) (-27.8098, -11.6279) knots 0 0 0 0 1 1 1 1
  spline S622 degree 3 poles (-27.8098, -11.6279) (-27.5516, -12.4583) (-27.4911, -12.5379) (-27.1185, -12.5379) knots 0 0 0 0 1 1 1 1
  spline S623 degree 3 poles (-27.1185, -12.5379) (-26.6213, -12.5379) (-26.6037, -12.4574) (-26.8925, -11.507) knots 0 0 0 0 1 1 1 1
  spline S624 degree 3 poles (-26.8925, -11.507) (-27.1406, -10.6905) (-27.6534, -8.6746) (-27.7356, -8.1923) knots 0 0 0 0 1 1 1 1
  spline S625 degree 3 poles (-27.7356, -8.1923) (-27.8182, -7.7078) (-27.761, -7.7232) (-29.8067, -7.6348) knots 0 0 0 0 1 1 1 1
  spline S626 degree 3 poles (-29.8067, -7.6348) (-30.827, -7.5907) (-31.9067, -7.5323) (-32.206, -7.505) knots 0 0 0 0 1 1 1 1
  spline S627 degree 3 poles (-32.206, -7.505) (-32.6776, -7.4619) (-32.7652, -7.4718) (-32.8624, -7.5793) knots 0 0 0 0 1 1 1 1
  spline S628 degree 3 poles (-32.8624, -7.5793) (-32.966, -7.6938) (-32.9548, -7.7695) (-32.717, -8.563) knots 0 0 0 0 1 1 1 1
  spline S629 degree 3 poles (-32.717, -8.563) (-32.2244, -10.2069) (-30.7953, -13.9852) (-30.6258, -14.0919) knots 0 0 0 0 1 1 1 1
  spline S630 degree 3 poles (-30.6258, -14.0919) (-30.4874, -14.179) (-29.6106, -14.3567) (-28.8266, -14.4565) knots 0 0 0 0 1 1 1 1
  spline S631 degree 3 poles (-28.8266, -14.4565) (-27.8326, -14.5831) (-27.8825, -14.5838) (-27.7547, -14.4426) knots 0 0 0 0 1 1 1 1
  spline S632 degree 3 poles (-17.6298, -13.7677) (-17.5645, -13.6891) (-17.592, -13.4603) (-17.7575, -12.7057) knots 0 0 0 0 1 1 1 1
  spline S633 degree 3 poles (-17.7575, -12.7057) (-17.9642, -11.7629) (-17.9658, -11.7403) (-17.8397, -11.5634) knots 0 0 0 0 1 1 1 1
  spline S634 degree 3 poles (-17.8397, -11.5634) (-17.5474, -11.1534) (-17.6489, -11.1668) (-15.2108, -11.2149) knots 0 0 0 0 1 1 1 1
  spline S635 degree 3 poles (-15.2108, -11.2149) (-13.2049, -11.2545) (-12.9582, -11.2473) (-12.8516, -11.146) knots 0 0 0 0 1 1 1 1
  spline S636 degree 3 poles (-12.8516, -11.146) (-12.742, -11.0418) (-12.7403, -10.9748) (-12.8299, -10.2978) knots 0 0 0 0 1 1 1 1
  spline S637 degree 3 poles (-12.8299, -10.2978) (-12.8834, -9.8935) (-12.9591, -9.2503) (-12.9981, -8.8685) knots 0 0 0 0 1 1 1 1
  spline S638 degree 3 poles (-12.9981, -8.8685) (-13.0379, -8.4788) (-13.1089, -8.1366) (-13.1598, -8.0883) knots 0 0 0 0 1 1 1 1
  spline S639 degree 3 poles (-13.1598, -8.0883) (-13.2265, -8.0253) (-13.9399, -7.9912) (-15.8408, -7.9602) knots 0 0 0 0 1 1 1 1
  spline S640 degree 3 poles (-15.8408, -7.9602) (-17.2654, -7.9369) (-19.4865, -7.8976) (-20.7767, -7.8728) knots 0 0 0 0 1 1 1 1
  spline S641 degree 3 poles (-20.7767, -7.8728) (-22.9185, -7.8315) (-23.1309, -7.8378) (-23.2197, -7.9448) knots 0 0 0 0 1 1 1 1
  spline S642 degree 3 poles (-23.2197, -7.9448) (-23.3036, -8.0459) (-23.2865, -8.2083) (-23.095, -9.1274) knots 0 0 0 0 1 1 1 1
  spline S643 degree 3 poles (-23.095, -9.1274) (-22.76, -10.7349) (-22.715, -10.8814) (-22.5286, -10.9746) knots 0 0 0 0 1 1 1 1
  spline S644 degree 3 poles (-22.5286, -10.9746) (-22.4295, -11.0241) (-21.9343, -11.0624) (-21.273, -11.0717) knots 0 0 0 0 1 1 1 1
  spline S645 degree 3 poles (-21.273, -11.0717) (-20.6724, -11.0802) (-20.0708, -11.0961) (-19.936, -11.1071) knots 0 0 0 0 1 1 1 1
  spline S646 degree 3 poles (-19.936, -11.1071) (-19.8013, -11.1181) (-19.628, -11.1297) (-19.551, -11.1328) knots 0 0 0 0 1 1 1 1
  spline S647 degree 3 poles (-19.551, -11.1328) (-19.474, -11.136) (-19.3234, -11.2093) (-19.2164, -11.2957) knots 0 0 0 0 1 1 1 1
  spline S648 degree 3 poles (-19.2164, -11.2957) (-19.0542, -11.4267) (-18.9825, -11.6043) (-18.7853, -12.3629) knots 0 0 0 0 1 1 1 1
  spline S649 degree 3 poles (-18.7853, -12.3629) (-18.5333, -13.3325) (-18.4326, -13.6344) (-18.3133, -13.7782) knots 0 0 0 0 1 1 1 1
  spline S650 degree 3 poles (-18.3133, -13.7782) (-18.2125, -13.8997) (-17.7332, -13.8923) (-17.6298, -13.7677) knots 0 0 0 0 1 1 1 1
  spline S651 degree 3 poles (31.6006, -12.5564) (31.6658, -12.4998) (31.7986, -12.2479) (31.8957, -11.9965) knots 0 0 0 0 1 1 1 1
  spline S652 degree 3 poles (31.8957, -11.9965) (32.033, -11.6412) (32.0557, -11.5086) (31.9978, -11.4004) knots 0 0 0 0 1 1 1 1
  spline S653 degree 3 poles (31.9978, -11.4004) (31.9301, -11.2738) (31.8778, -11.2655) (31.4227, -11.3093) knots 0 0 0 0 1 1 1 1
  spline S654 degree 3 poles (31.4227, -11.3093) (31.1474, -11.3358) (30.8804, -11.3981) (30.8295, -11.4478) knots 0 0 0 0 1 1 1 1
  spline S655 degree 3 poles (30.8295, -11.4478) (30.7786, -11.4974) (30.6607, -11.7481) (30.5675, -12.0048) knots 0 0 0 0 1 1 1 1
  spline S656 degree 3 poles (30.5675, -12.0048) (30.4293, -12.3854) (30.4136, -12.4962) (30.4819, -12.6057) knots 0 0 0 0 1 1 1 1
  spline S657 degree 3 poles (30.4819, -12.6057) (30.5554, -12.7234) (30.6226, -12.735) (31.024, -12.6996) knots 0 0 0 0 1 1 1 1
  spline S658 degree 3 poles (31.024, -12.6996) (31.276, -12.6774) (31.5355, -12.613) (31.6006, -12.5564) knots 0 0 0 0 1 1 1 1
  spline S659 degree 3 poles (-5.701, -11.2196) (-5.5885, -11.0954) (-5.5854, -10.9804) (-5.6588, -9.659) knots 0 0 0 0 1 1 1 1
  spline S660 degree 3 poles (-5.6588, -9.659) (-5.7079, -8.7757) (-5.769, -8.2012) (-5.8191, -8.1502) knots 0 0 0 0 1 1 1 1
  spline S661 degree 3 poles (-5.8191, -8.1502) (-5.8774, -8.0909) (-6.7654, -8.0548) (-8.9814, -8.0215) knots 0 0 0 0 1 1 1 1
  spline S662 degree 3 poles (-8.9814, -8.0215) (-11.9164, -7.9773) (-12.0682, -7.9813) (-12.1782, -8.1038) knots 0 0 0 0 1 1 1 1
  spline S663 degree 3 poles (-12.1782, -8.1038) (-12.2857, -8.2235) (-12.2846, -8.3134) (-12.1624, -9.3876) knots 0 0 0 0 1 1 1 1
  spline S664 degree 3 poles (-12.1624, -9.3876) (-12.0047, -10.7737) (-11.9682, -11.004) (-11.8848, -11.1391) knots 0 0 0 0 1 1 1 1
  spline S665 degree 3 poles (-11.8848, -11.1391) (-11.819, -11.2456) (-11.8803, -11.2432) (-6.9463, -11.3332) knots 0 0 0 0 1 1 1 1
  spline S666 degree 3 poles (-6.9463, -11.3332) (-5.9129, -11.3521) (-5.8125, -11.3429) (-5.701, -11.2196) knots 0 0 0 0 1 1 1 1
  spline S667 degree 3 poles (3.2413, -11.2356) (3.3378, -11.1193) (3.3821, -10.232) (3.4735, -6.5874) knots 0 0 0 0 1 1 1 1
  spline S668 degree 3 poles (3.4735, -6.5874) (3.5614, -3.0789) (3.55, -1.1919) (3.4406, -1.1226) knots 0 0 0 0 1 1 1 1
  spline S669 degree 3 poles (3.4406, -1.1226) (3.3855, -1.0878) (2.3077, -1.0588) (1.0455, -1.0582) knots 0 0 0 0 1 1 1 1
  spline S670 degree 3 poles (1.0455, -1.0582) (-0.9884, -1.0572) (-1.2541, -1.0697) (-1.292, -1.1684) knots 0 0 0 0 1 1 1 1
  spline S671 degree 3 poles (-1.292, -1.1684) (-1.3375, -1.287) (-1.3475, -2.4527) (-1.3273, -5.3049) knots 0 0 0 0 1 1 1 1
  spline S672 degree 3 poles (-1.3273, -5.3049) (-1.3168, -6.8026) (-1.2984, -7.084) (-1.2049, -7.1775) knots 0 0 0 0 1 1 1 1
  spline S673 degree 3 poles (-1.2049, -7.1775) (-1.1225, -7.2599) (-0.9486, -7.2875) (-0.512, -7.2875) knots 0 0 0 0 1 1 1 1
  spline S674 degree 3 poles (-0.512, -7.2875) (0.0225, -7.2875) (0.0888, -7.3033) (0.288, -7.4781) knots 0 0 0 0 1 1 1 1
  line L65 (0.288, -7.4781) -> (0.5052, -7.6687)
  line L66 (0.5052, -7.6687) -> (0.5052, -9.3802)
  spline S675 degree 3 poles (0.5052, -9.3802) (0.5052, -10.8745) (0.5199, -11.1079) (0.6211, -11.2197) knots 0 0 0 0 1 1 1 1
  spline S676 degree 3 poles (0.6211, -11.2197) (0.7248, -11.3343) (0.8635, -11.3477) (1.9426, -11.3477) knots 0 0 0 0 1 1 1 1
  spline S677 degree 3 poles (1.9426, -11.3477) (2.9628, -11.3477) (3.1625, -11.3305) (3.2413, -11.2356) knots 0 0 0 0 1 1 1 1
  spline S678 degree 3 poles (13.8596, -11.2396) (14.0049, -11.1932) (14.0613, -10.9546) (14.2608, -9.5422) knots 0 0 0 0 1 1 1 1
  spline S679 degree 3 poles (14.2608, -9.5422) (14.4151, -8.4499) (14.4344, -8.1749) (14.363, -8.0888) knots 0 0 0 0 1 1 1 1
  spline S680 degree 3 poles (14.363, -8.0888) (14.2871, -7.9974) (13.9396, -7.9837) (11.8615, -7.9903) knots 0 0 0 0 1 1 1 1
  line L67 (11.8615, -7.9903) -> (9.4482, -7.998)
  line L68 (9.4482, -7.998) -> (9.2086, -7.7658)
  line L69 (9.2086, -7.7658) -> (8.9691, -7.5336)
  line L70 (8.9691, -7.5336) -> (9.0096, -7.008)
  spline S681 degree 3 poles (9.0096, -7.008) (9.0319, -6.7189) (9.0797, -5.8382) (9.1157, -5.0509) knots 0 0 0 0 1 1 1 1
  line L71 (9.1157, -5.0509) -> (9.1813, -3.6194)
  line L72 (9.1813, -3.6194) -> (9.376, -3.428)
  line L73 (9.376, -3.428) -> (9.5708, -3.2367)
  line L74 (9.5708, -3.2367) -> (12.3359, -3.1891)
  line L75 (12.3359, -3.1891) -> (15.1011, -3.1415)
  line L76 (15.1011, -3.1415) -> (15.3389, -3.3908)
  line L77 (15.3389, -3.3908) -> (15.5766, -3.6401)
  line L78 (15.5766, -3.6401) -> (15.539, -4.1889)
  spline S682 degree 3 poles (15.539, -4.1889) (15.4906, -4.896) (15.5446, -4.9773) (16.0628, -4.9773) knots 0 0 0 0 1 1 1 1
  spline S683 degree 3 poles (16.0628, -4.9773) (16.2948, -4.9773) (16.4793, -4.9409) (16.5248, -4.8861) knots 0 0 0 0 1 1 1 1
  spline S684 degree 3 poles (16.5248, -4.8861) (16.6673, -4.7143) (16.8463, -1.3396) (16.7232, -1.1446) knots 0 0 0 0 1 1 1 1
  spline S685 degree 3 poles (16.7232, -1.1446) (16.6798, -1.0759) (15.5646, -1.0571) (11.5318, -1.0571) knots 0 0 0 0 1 1 1 1
  spline S686 degree 3 poles (11.5318, -1.0571) (6.9558, -1.0571) (6.3836, -1.0691) (6.2856, -1.1671) knots 0 0 0 0 1 1 1 1
  spline S687 degree 3 poles (6.2856, -1.1671) (6.1921, -1.2605) (6.1753, -1.5161) (6.1741, -2.8647) knots 0 0 0 0 1 1 1 1
  spline S688 degree 3 poles (6.1741, -2.8647) (6.1725, -4.5926) (6.1533, -5.2164) (5.9924, -8.7897) knots 0 0 0 0 1 1 1 1
  spline S689 degree 3 poles (5.9924, -8.7897) (5.8941, -10.97) (5.8946, -11.1739) (5.9978, -11.2494) knots 0 0 0 0 1 1 1 1
  spline S690 degree 3 poles (5.9978, -11.2494) (6.0821, -11.311) (7.0724, -11.3237) (9.9407, -11.2998) knots 0 0 0 0 1 1 1 1
  spline S691 degree 3 poles (9.9407, -11.2998) (12.0474, -11.2823) (13.8109, -11.2552) (13.8596, -11.2396) knots 0 0 0 0 1 1 1 1
  spline S692 degree 3 poles (17.5345, -11.0852) (17.6901, -10.9118) (18.1306, -8.2294) (18.0298, -8.0692) knots 0 0 0 0 1 1 1 1
  spline S693 degree 3 poles (18.0298, -8.0692) (17.9725, -7.978) (17.8253, -7.9481) (17.3555, -7.9323) knots 0 0 0 0 1 1 1 1
  line L79 (17.3555, -7.9323) -> (16.7544, -7.9122)
  line L80 (16.7544, -7.9122) -> (16.5452, -7.6277)
  spline S694 degree 3 poles (16.5452, -7.6277) (16.4302, -7.4713) (16.3498, -7.3071) (16.3666, -7.2629) knots 0 0 0 0 1 1 1 1
  spline S695 degree 3 poles (16.3666, -7.2629) (16.3834, -7.2187) (16.424, -6.9147) (16.457, -6.5874) knots 0 0 0 0 1 1 1 1
  spline S696 degree 3 poles (16.457, -6.5874) (16.5372, -5.7893) (16.5008, -5.7474) (15.7275, -5.7474) knots 0 0 0 0 1 1 1 1
  spline S697 degree 3 poles (15.7275, -5.7474) (15.1509, -5.7474) (15.1505, -5.7472) (14.9253, -5.4908) knots 0 0 0 0 1 1 1 1
  spline S698 degree 3 poles (14.9253, -5.4908) (14.7006, -5.2348) (14.7001, -5.2328) (14.7484, -4.6798) knots 0 0 0 0 1 1 1 1
  spline S699 degree 3 poles (14.7484, -4.6798) (14.791, -4.1909) (14.7816, -4.1141) (14.6689, -4.0286) knots 0 0 0 0 1 1 1 1
  spline S700 degree 3 poles (14.6689, -4.0286) (14.5667, -3.9512) (14.1167, -3.9313) (12.428, -3.9295) knots 0 0 0 0 1 1 1 1
  spline S701 degree 3 poles (12.428, -3.9295) (11.2343, -3.9282) (10.2376, -3.9566) (10.1373, -3.9948) knots 0 0 0 0 1 1 1 1
  spline S702 degree 3 poles (10.1373, -3.9948) (9.9119, -4.0805) (9.9024, -4.1333) (9.8484, -5.6064) knots 0 0 0 0 1 1 1 1
  spline S703 degree 3 poles (9.8484, -5.6064) (9.8238, -6.2797) (9.7887, -6.8546) (9.7706, -6.8839) knots 0 0 0 0 1 1 1 1
  spline S704 degree 3 poles (9.7706, -6.8839) (9.7525, -6.9132) (9.7847, -7.0044) (9.8422, -7.0864) knots 0 0 0 0 1 1 1 1
  spline S705 degree 3 poles (9.8422, -7.0864) (9.9458, -7.2344) (9.9685, -7.2356) (12.3864, -7.2225) knots 0 0 0 0 1 1 1 1
  line L81 (12.3864, -7.2225) -> (14.8262, -7.2094)
  line L82 (14.8262, -7.2094) -> (15.0423, -7.4784)
  line L83 (15.0423, -7.4784) -> (15.2585, -7.7474)
  line L84 (15.2585, -7.7474) -> (15.091, -9.04)
  spline S706 degree 3 poles (15.091, -9.04) (14.9989, -9.751) (14.9041, -10.4817) (14.8802, -10.6639) knots 0 0 0 0 1 1 1 1
  spline S707 degree 3 poles (14.8802, -10.6639) (14.8099, -11.2012) (14.826, -11.2077) (16.2189, -11.2077) knots 0 0 0 0 1 1 1 1
  spline S708 degree 3 poles (16.2189, -11.2077) (17.2786, -11.2077) (17.4379, -11.1929) (17.5345, -11.0852) knots 0 0 0 0 1 1 1 1
  spline S709 degree 3 poles (19.3627, -10.9802) (19.5005, -10.7622) (19.9287, -8.3357) (19.8704, -8.1034) knots 0 0 0 0 1 1 1 1
  spline S710 degree 3 poles (19.8704, -8.1034) (19.8272, -7.9313) (19.796, -7.9175) (19.4509, -7.9175) knots 0 0 0 0 1 1 1 1
  spline S711 degree 3 poles (19.4509, -7.9175) (19.1818, -7.9175) (19.0494, -7.9516) (18.9749, -8.04) knots 0 0 0 0 1 1 1 1
  spline S712 degree 3 poles (18.9749, -8.04) (18.9143, -8.1119) (18.7773, -8.7354) (18.6433, -9.5485) knots 0 0 0 0 1 1 1 1
  spline S713 degree 3 poles (18.6433, -9.5485) (18.3819, -11.1339) (18.3826, -11.1377) (18.9233, -11.1377) knots 0 0 0 0 1 1 1 1
  spline S714 degree 3 poles (18.9233, -11.1377) (19.1996, -11.1377) (19.2818, -11.1082) (19.3627, -10.9802) knots 0 0 0 0 1 1 1 1
  spline S715 degree 3 poles (21.1502, -10.9703) (21.3462, -10.7342) (21.9876, -7.0831) (22.2106, -4.9341) knots 0 0 0 0 1 1 1 1
  spline S716 degree 3 poles (22.2106, -4.9341) (22.314, -3.9381) (22.276, -3.844) (21.7799, -3.8666) knots 0 0 0 0 1 1 1 1
  spline S717 degree 3 poles (21.7799, -3.8666) (21.2376, -3.8914) (21.1769, -3.9663) (21.1217, -4.6794) knots 0 0 0 0 1 1 1 1
  spline S718 degree 3 poles (21.1217, -4.6794) (21.0422, -5.7081) (20.7435, -7.9562) (20.5193, -9.2126) knots 0 0 0 0 1 1 1 1
  spline S719 degree 3 poles (20.5193, -9.2126) (20.214, -10.9244) (20.2177, -10.8889) (20.3328, -11.0041) knots 0 0 0 0 1 1 1 1
  spline S720 degree 3 poles (20.3328, -11.0041) (20.4532, -11.1245) (21.0424, -11.1001) (21.1502, -10.9703) knots 0 0 0 0 1 1 1 1
  spline S721 degree 3 poles (31.9572, -10.4715) (32.1795, -10.4437) (32.3933, -10.3728) (32.4511, -10.3076) knots 0 0 0 0 1 1 1 1
  spline S722 degree 3 poles (32.4511, -10.3076) (32.5508, -10.1951) (32.8276, -9.3446) (33.1245, -8.2381) knots 0 0 0 0 1 1 1 1
  spline S723 degree 3 poles (33.1245, -8.2381) (33.2595, -7.7354) (33.2631, -7.6734) (33.164, -7.5743) knots 0 0 0 0 1 1 1 1
  spline S724 degree 3 poles (33.164, -7.5743) (33.0186, -7.4288) (32.0985, -7.4599) (31.9236, -7.6161) knots 0 0 0 0 1 1 1 1
  spline S725 degree 3 poles (31.9236, -7.6161) (31.8584, -7.6744) (31.7544, -7.9472) (31.6925, -8.2223) knots 0 0 0 0 1 1 1 1
  spline S726 degree 3 poles (31.6925, -8.2223) (31.6307, -8.4974) (31.4871, -9.0461) (31.3736, -9.4416) knots 0 0 0 0 1 1 1 1
  spline S727 degree 3 poles (31.3736, -9.4416) (31.26, -9.837) (31.1671, -10.2214) (31.1671, -10.2956) knots 0 0 0 0 1 1 1 1
  spline S728 degree 3 poles (31.1671, -10.2956) (31.1671, -10.4396) (31.3615, -10.5916) (31.4887, -10.5472) knots 0 0 0 0 1 1 1 1
  spline S729 degree 3 poles (31.4887, -10.5472) (31.5308, -10.5325) (31.7416, -10.4985) (31.9572, -10.4715) knots 0 0 0 0 1 1 1 1
  spline S730 degree 3 poles (5.1437, -8.8451) (5.2357, -8.7424) (5.2667, -8.3138) (5.335, -6.2024) knots 0 0 0 0 1 1 1 1
  spline S731 degree 3 poles (5.335, -6.2024) (5.3797, -4.8163) (5.4061, -3.0995) (5.3934, -2.3872) knots 0 0 0 0 1 1 1 1
  line L85 (5.3934, -2.3872) -> (5.3705, -1.0921)
  line L86 (5.3705, -1.0921) -> (4.9155, -1.0722)
  spline S732 degree 3 poles (4.9155, -1.0722) (4.525, -1.0551) (4.4483, -1.0719) (4.3748, -1.1908) knots 0 0 0 0 1 1 1 1
  spline S733 degree 3 poles (4.3748, -1.1908) (4.313, -1.2908) (4.2856, -1.9112) (4.2768, -3.4159) knots 0 0 0 0 1 1 1 1